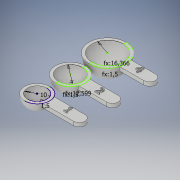
# Autodesk Inventor part: Pigmentlöffel
Saved by Autodesk Inventor 2018 (Build 220112000, 112)
## iProperties
Created: 2018-01-23
Part Number: Pigmentlöffel
Material: Generisch
Document SubType Name: Modeling
Designer: JochenAlt
Density: 1 g/cm^3
Appearance: Vorgabe
Author: JochenAlt
Autodesk Inventor part; units mm, degrees
ref_plane "XZ Plane" through (0, 0, 0) normal (0, 1, 0) x (-1, 0, 0)
ref_plane "XY Plane" through (0, 0, 0) normal (0, 0, 1) x (1, 0, 0)
sketch "Skizze1" plane through (0, 0, 0) normal (0, 0, 1) x (1, 0, 0)
  arc A0 (0, -5) -> (0, 5) centre (0, 0) ccw
  arc A1 (0, -6.5) -> (0, 6.5) centre (0, 0) ccw
  line L0 (0, -6.5) -> (0, -5)
  line L1 (0, 5) -> (0, 6.5)
  arc A2 (0, 11.07) -> (0, 23.669) centre (0, 17.3695) ccw
  arc A3 (0, 9.57) -> (0, 25.169) centre (0, 17.3695) ccw
  arc A4 (0, 28.5978) -> (0, 44.9639) centre (0, 36.7809) ccw
  arc A5 (0, 27.0978) -> (0, 46.4639) centre (0, 36.7809) ccw
  line L2 (0, 44.9639) -> (0, 46.4639)
  line L3 (0, 27.0978) -> (0, 28.5978)
  line L4 (0, 9.57) -> (0, 11.07)
  line L5 (0, 23.669) -> (0, 25.169)
  dimension "d0" = 10
  dimension "d8" = 1.5
  dimension "d9" = 12.599
  dimension "d10" = 1.5
  dimension "d11" = 16.3661
  dimension "d12" = 1.5
  constraints: 12 end point, 12 point on circle, 6 centre point, 6 vertical, 4 coincident
  measures "d0" diameter of A0
  measures "d8" radial gap between concentric circles of A1 A0
  measures "d9" diameter of A2
  measures "d10" radial gap between concentric circles of A3 A2
  measures "d11" diameter of A4
  measures "d12" radial gap between concentric circles of A5 A4
revolve "Umdrehung1" add sketch "Skizze1" angle 180 about axis through (0, -6.5, 0) along (0, 1, 0) contours A0 L1 A1 L0
revolve "Umdrehung2" add sketch "Skizze1" angle 180 about axis through (0, 9.57, 0) along (0, 1, 0) contours A2 L5 A3 L4
revolve "Umdrehung3" add sketch "Skizze1" angle 180 about axis through (0, 27.0978, 0) along (0, 1, 0) contours A4 L2 A5 L3
ref_plane "Arbeitsebene1" through (25, 0, 0) normal (1, 0, 0) x (0, 1, 0)
sketch "Skizze3" plane through (25, 0, 0) normal (1, 0, 0) x (0, 1, 0)
  line L0 (-5, 0) -> (5, 0) projected
  line L1 (-3, 0) -> (3, 0)
  line L2 (3, 0) -> (3, -2)
  line L3 (3, -2) -> (-3, -2)
  line L4 (-3, -2) -> (-3, 0)
  line L5 (14.3695, 0) -> (20.3695, 0)
  line L6 (20.3695, 0) -> (20.3695, -2)
  line L7 (20.3695, -2) -> (14.3695, -2)
  line L8 (14.3695, -2) -> (14.3695, 0)
  line L9 (33.7809, 0) -> (39.7809, 0)
  line L10 (39.7809, 0) -> (39.7809, -2)
  line L11 (39.7809, -2) -> (33.7809, -2)
  line L12 (33.7809, -2) -> (33.7809, 0)
  line L13 (25.169, 0) -> (9.57, 0) construction
  line L14 (46.4639, 0) -> (27.0978, 0) construction
  arc A0 (-5, 0) -> (5, 0) centre (0, 0) ccw construction
  line L15 (6.5, 0) -> (-6.5, 0) construction
  line L16 (0, 1.9366) -> (0, -11.6197) construction
  line L17 (-17.0928, 0) -> (57.0567, 0) construction
  line L18 (36.7809, 0) -> (36.7809, -9.6771) construction
  line L19 (17.3695, 0) -> (17.3695, -7.848) construction
  dimension "d16" = 2
  dimension "d17" = 6
  dimension "d21" = 6
  dimension "d22" = 6
  constraints: 28 end point, 6 parallel, 3 coincident, 3 horizontal, 3 perpendicular, 3 point on line, 2 collinear, 2 vertical, 4 other
  measures "d16" distance of the line from the sketch origin of L3
  measures "d17" distance between parallel lines of L2 L4
  measures "d21" distance between parallel lines of L6 L8
  measures "d22" distance between parallel lines of L10 L12
extrude "Extrusion2" add sketch "Skizze3" against normal up to next
fillet "Rundung1" radius 3 6 edges at (25, 3, -1) (25, -3, -1) (25, 14.3695, -1) (25, 20.3695, -1) (25, 33.7809, -1) (25, 39.7809, -1)
sketch "Skizze5" plane through (0, 0, 0) normal (0, 0, 1) x (1, 0, 0)
  line L0 (14.4706, 2.3985) -> (25.3002, 2.3985) construction
  line L1 (25.3002, 2.3985) -> (25.3002, -2.3176) construction
  line L2 (25.3002, -2.3176) -> (14.4706, -2.3176) construction
  line L3 (14.4706, -2.3176) -> (14.4706, 2.3985) construction
  line L4 (14.2377, 19.2833) -> (24.5433, 19.2833) construction
  line L5 (24.5433, 19.2833) -> (24.5433, 14.5672) construction
  line L6 (24.5433, 14.5672) -> (14.2377, 14.5672) construction
  line L7 (14.2377, 14.5672) -> (14.2377, 19.2833) construction
  line L8 (14.82, 39.021) -> (28.6189, 39.021) construction
  line L9 (28.6189, 39.021) -> (28.6189, 34.0138) construction
  line L10 (28.6189, 34.0138) -> (14.82, 34.0138) construction
  line L11 (14.82, 34.0138) -> (14.82, 39.021) construction
  line L12 (16.7085, -1.1128) -> (15.001, -1.1128)
  line L13 (15.001, -1.1128) -> (15.001, -0.7555)
  line L14 (15.001, -0.7555) -> (15.6363, -0.7555)
  line L15 (15.6363, -0.7555) -> (15.6363, 1.5902)
  line L16 (15.6363, 1.5902) -> (15.001, 1.5902)
  line L17 (15.001, 1.5902) -> (15.001, 1.9107)
  spline S0 degree 2 poles (15.001, 1.9107) (15.3612, 1.9107) (15.7016, 2.1149) (15.7243, 2.3985) knots 0 0 0 1 2 2 2
  line L18 (15.7243, 2.3985) -> (16.0873, 2.3985)
  line L19 (16.0873, 2.3985) -> (16.0873, -0.7555)
  line L20 (16.0873, -0.7555) -> (16.7085, -0.7555)
  line L21 (16.7085, -0.7555) -> (16.7085, -1.1128)
  line L22 (16.6514, 15.7095) -> (14.493, 15.7095)
  line L23 (14.493, 15.7095) -> (14.493, 16.2059)
  spline S1 degree 2 poles (14.493, 16.2059) (14.7256, 16.4243) (15.1397, 16.8299) (15.3382, 17.0483) knots 0 0 0 1 2 2 2
  spline S2 degree 2 poles (15.3382, 17.0483) (15.7381, 17.4879) (16.0303, 18.0155) (16.0303, 18.2963) knots 0 0 0 1 2 2 2
  spline S3 degree 2 poles (16.0303, 18.2963) (16.0303, 18.4437) (15.9395, 18.665) (15.8572, 18.7359) knots 0 0 0 1 2 2 2
  spline S4 degree 2 poles (15.8572, 18.7359) (15.775, 18.8068) (15.5594, 18.8777) (15.429, 18.8777) knots 0 0 0 1 2 2 2
  spline S5 degree 2 poles (15.429, 18.8777) (15.3042, 18.8777) (15.0489, 18.8153) (14.9326, 18.7671) knots 0 0 0 1 2 2 2
  spline S6 degree 2 poles (14.9326, 18.7671) (14.8333, 18.7274) (14.649, 18.6139) (14.5923, 18.5742) knots 0 0 0 1 2 2 2
  line L24 (14.5923, 18.5742) -> (14.5667, 18.5742)
  line L25 (14.5667, 18.5742) -> (14.5667, 19.0734)
  spline S7 degree 2 poles (14.5667, 19.0734) (14.7114, 19.1443) (15.2304, 19.2833) (15.463, 19.2833) knots 0 0 0 1 2 2 2
  spline S8 degree 2 poles (15.463, 19.2833) (15.9537, 19.2833) (16.5068, 18.7642) (16.5068, 18.3218) knots 0 0 0 1 2 2 2
  spline S9 degree 2 poles (16.5068, 18.3218) (16.5068, 18.1147) (16.4103, 17.7687) (16.3252, 17.6212) knots 0 0 0 1 2 2 2
  spline S10 degree 2 poles (16.3252, 17.6212) (16.2401, 17.4681) (15.9934, 17.1674) (15.8572, 17.0228) knots 0 0 0 1 2 2 2
  spline S11 degree 2 poles (15.8572, 17.0228) (15.636, 16.7817) (15.0943, 16.2655) (14.9326, 16.1151) knots 0 0 0 1 2 2 2
  line L26 (14.9326, 16.1151) -> (16.6514, 16.1151)
  line L27 (16.6514, 16.1151) -> (16.6514, 15.7095)
  line L28 (17.3272, 36.7236) -> (16.9103, 36.7236)
  line L29 (16.9103, 36.7236) -> (16.9103, 35.521)
  line L30 (16.9103, 35.521) -> (16.4593, 35.521)
  line L31 (16.4593, 35.521) -> (16.4593, 36.7236)
  line L32 (16.4593, 36.7236) -> (14.9135, 36.7236)
  line L33 (14.9135, 36.7236) -> (14.9135, 37.2171)
  line L34 (14.9135, 37.2171) -> (16.4792, 39.021)
  line L35 (16.4792, 39.021) -> (16.9103, 39.021)
  line L36 (16.9103, 39.021) -> (16.9103, 37.1008)
  line L37 (16.9103, 37.1008) -> (17.3272, 37.1008)
  line L38 (17.3272, 37.1008) -> (17.3272, 36.7236)
  line L39 (16.4593, 37.1008) -> (16.4593, 38.4679)
  line L40 (16.4593, 38.4679) -> (15.2823, 37.1008)
  line L41 (15.2823, 37.1008) -> (16.4593, 37.1008)
  point P0 (0, 0)
  constraints: 6 other
extrude "Extrusion3" add sketch "Skizze5" along normal blind 0.6
equation "\"d9\" = 1.2599 * d0"
equation "\"d10\" = d8"
equation "\"d11\" = 1.299 * d9"
equation "\"d12\" = d10"
equation "\"d21\" = d17"
equation "\"d22\" = d17"
